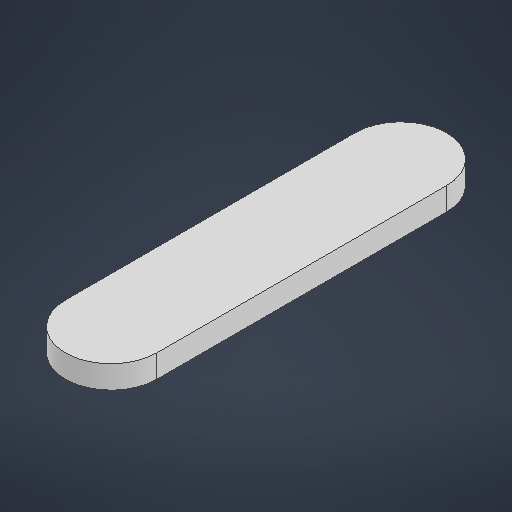
# Autodesk Inventor part: 连杆1
Saved by Autodesk Inventor 2025 (Build 290162000, 162)
## iProperties
Created: 2025-11-07
Part Number: 连杆1
Material: 常规
Document SubType Name: Modeling
Designer: XH
Density: 1 g/cm^3
Appearance: 默认
Author: XH
Autodesk Inventor part; units mm, degrees
ref_plane "YZ Plane" through (0, 0, 0) normal (1, 0, 0) x (0, 1, 0)
ref_plane "XZ Plane" through (0, 0, 0) normal (0, 1, 0) x (-1, 0, 0)
ref_plane "XY Plane" through (0, 0, 0) normal (0, 0, 1) x (1, 0, 0)
sketch "草图1" plane through (0, 0, 0) normal (0, 1, 0) x (-1, 0, 0)
  line L0 (0, 0) -> (0, -50) construction
  line L1 (-6, -6) -> (-6, -44)
  line L2 (6, -44) -> (6, -6)
  arc A0 (6, -6) -> (-6, -6) centre (0, -6) ccw
  arc A1 (-6, -44) -> (6, -44) centre (0, -44) ccw
  point P0 (0, -25)
  dimension "d0" = 50
  dimension "d1" = 6
  constraints: 8 end point, 6 point on circle, 4 tangent, 2 centre point, 2 point on line, 1 midpoint, 1 parallel, 1 vertical
  measures "d0" distance of L0.start L0.end
  measures "d1" radius of A0
extrude "拉伸1" add sketch "草图1" along normal blind 3
